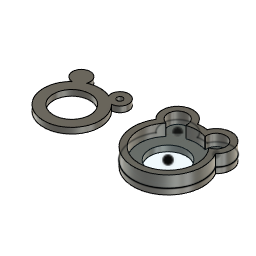
PushPop (Autodesk Fusion 360 design; units mm, degrees)
Autodesk Fusion 360 part; units mm, degrees
sketch "スケッチ1" plane through (0, 0, 0) normal (0, 0, 1) x (1, 0, 0)
  circle A0 centre (0, 0) radius 9.5
  circle A1 centre (0, 0) radius 15
  circle A2 centre (-10, 15) radius 5
  circle A3 centre (10, 15) radius 5
  dimension "d1" = 19
  constraint coincident A0.centre A1.centre
  measures "d1" diameter of A0
extrude "押し出し1" add sketch "スケッチ1" along normal blind 3 makes body 1
copy_body "ボディのコピーと貼り付け1" bodies 1 makes body 2
move_body "移動1" bodies 2 to x (1, 0, 0) y (0, 1, 0) z (0, 0, 1) at (50, 0, 0)
sketch "スケッチ2" plane through (0, 0, 3) normal (0, 0, 1) x (-1, 0, 0)
  circle A0 centre (-50, 0) radius 9.5
  arc A1 (-61.0747, -10.1169) -> (-55.0791, -14.1139) centre (-60, -15) ccw
  arc A2 (-55.0791, -14.1139) -> (-44.9209, -14.1139) centre (-50, 0) ccw
  arc A3 (-44.9209, -14.1139) -> (-38.9253, -10.1169) centre (-40, -15) ccw
  arc A4 (-38.9253, -10.1169) -> (-61.0747, -10.1169) centre (-50, 0) ccw
  arc A5 (-52.5148, -17.8235) -> (-47.4852, -17.8235) centre (-50, 0) ccw
  arc A6 (-47.4852, -17.8235) -> (-34.5148, -9.1765) centre (-40, -15) ccw
  arc A7 (-34.5148, -9.1765) -> (-65.4852, -9.1765) centre (-50, 0) ccw
  arc A8 (-65.4852, -9.1765) -> (-52.5148, -17.8235) centre (-60, -15) ccw
  dimension "d4" = 3
extrude "押し出し2" add sketch "スケッチ2" along normal blind 3 contours A5 A6 A7 A8 bodies 2
extrude "押し出し3" add 1 faces at (63.6616, 9.5234, 3) along direction (0, 0, -1) blind 3 on bodies 2 bodies 2
extrude "押し出し4" add 1 faces at (63.6616, 9.5234, 6) along direction (0, 0, 1) blind 3 on bodies 2 bodies 2
sketch "スケッチ3" plane through (0, 0, 3) normal (0, 0, 1) x (-1, 0, 0)
  circle A0 centre (0, 0) radius 9.5
  arc A1 (-11.0747, -10.1169) -> (-5.0791, -14.1139) centre (-10, -15) ccw
  arc A2 (-5.0791, -14.1139) -> (5.0791, -14.1139) centre (0, 0) ccw
  arc A3 (5.0791, -14.1139) -> (11.0747, -10.1169) centre (10, -15) ccw
  arc A4 (11.0747, -10.1169) -> (-11.0747, -10.1169) centre (0, 0) ccw
  circle A5 centre (-10, -15) radius 1.5
  circle A6 centre (-60, -15) radius 1.5
  arc A7 (10.2406, -10.4063) -> (-10.2406, -10.4063) centre (0, 0) ccw
  arc A8 (-10.2406, -10.4063) -> (-5.6671, -13.4552) centre (-10, -15) ccw
  arc A9 (-5.6671, -13.4552) -> (5.6671, -13.4552) centre (0, 0) ccw
  arc A10 (5.6671, -13.4552) -> (10.2406, -10.4063) centre (10, -15) ccw
  dimension "d11" = 3
  dimension "d12" = 3
  dimension "d19" = -0.4
  constraint concentric A1 A5
  measures "d11" diameter of A5
  measures "d12" diameter of A6
extrude "押し出し5" cut sketch "スケッチ3" against normal blind 11 contours A6 bodies 2
extrude "押し出し6" cut sketch "スケッチ3" against normal blind 10 contours A5 bodies 1
sketch "スケッチ4" plane through (0, 0, 9) normal (0, 0, 1) x (-1, 0, 0)
  arc A0 (-38.9253, -10.1169) -> (-61.0747, -10.1169) centre (-50, 0) ccw
  arc A1 (-44.9209, -14.1139) -> (-38.9253, -10.1169) centre (-40, -15) ccw
  arc A2 (-55.0791, -14.1139) -> (-44.9209, -14.1139) centre (-50, 0) ccw
  arc A3 (-61.0747, -10.1169) -> (-55.0791, -14.1139) centre (-60, -15) ccw
  arc A4 (-65.4852, -9.1765) -> (-52.5148, -17.8235) centre (-60, -15) ccw
  arc A5 (-52.5148, -17.8235) -> (-47.4852, -17.8235) centre (-50, 0) ccw
  arc A6 (-47.4852, -17.8235) -> (-34.5148, -9.1765) centre (-40, -15) ccw
  arc A7 (-34.5148, -9.1765) -> (-65.4852, -9.1765) centre (-50, 0) ccw
  circle A8 centre (-38.9253, -10.1169) radius 0.1872
  circle A9 centre (-61.0747, -10.1169) radius 0.2046
  circle A10 centre (-55.0791, -14.1139) radius 0.2488
  circle A11 centre (-44.9209, -14.1139) radius 0.2346
  constraint coincident A0.start A1.end
  constraint coincident A0.end A3.start
  constraint coincident A2.start A3.end
  constraint coincident A1.start A2.end
extrude "押し出し7" cut sketch "スケッチ4" against normal blind 6 contours A0 A1 A8 | A0 A3 A9 | A1 A2 A11 | A1 A2 A11 | A2 A3 A10 picked at (-38.7969, -10.0783) picked at (-61.2147, -10.0734) picked at (-54.9651, -14.2507) bodies 2
extrude "押し出し8" cut sketch "スケッチ3" against normal blind 4 contours A1 A2 A3 A4 bodies 1
